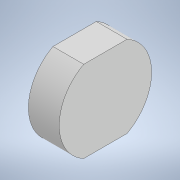
# Autodesk Inventor part: 711117
Saved by Autodesk Inventor 2022 (Build 260153000, 153)
## iProperties
Created: 2021-10-21
Part Number: 711117
Material: Типовые
Document SubType Name: Modeling
Designer: RaNSiD
Density: 1 g/cm^3
Appearance: По умолчанию
Author: RaNSiD
Autodesk Inventor part; units mm, degrees
ref_plane "YZ Plane" through (0, 0, 0) normal (1, 0, 0) x (0, 1, 0)
ref_plane "XZ Plane" through (0, 0, 0) normal (0, 1, 0) x (-1, 0, 0)
ref_plane "XY Plane" through (0, 0, 0) normal (0, 0, 1) x (1, 0, 0)
sketch "Эскиз1" plane through (0, 0, 0) normal (0, 0, 1) x (1, 0, 0)
  line L0 (0, 0) -> (20, 0)
  line L1 (20, 0) -> (20, 30)
  line L2 (20, 30) -> (0, 30)
  line L3 (0, 30) -> (0, 0)
  dimension "d0" = 20
  dimension "d1" = 30
  constraints: 8 end point, 2 parallel, 1 horizontal, 1 perpendicular
  measures "d0" distance of L2.end L1.end
  measures "d1" distance of L1.end L0.end
revolve "Вращение1" add sketch "Эскиз1" angle 360 about axis through (0, 0, 0) along (1, 0, 0)
sketch "Эскиз2" plane through (0, 0, 0) normal (0, 0, 1) x (1, 0, 0)
  line L0 (0, -30) -> (0, 30) construction
  line L1 (0, 20.647) -> (0, 23.353)
  line L2 (0, 23.353) -> (4, 24.5)
  line L3 (4, 24.5) -> (4, 19.5)
  line L4 (4, 19.5) -> (0, 20.647)
  line L5 (4, 22) -> (0, 22) construction
  line L6 (0, 0) -> (20.0289, 0)
  dimension "d3" = 74
  dimension "d4" = 74
  dimension "d5" = 5
  dimension "d6" = 4
  dimension "d7" = 22
  constraints: 12 end point, 2 midpoint, 2 point on line, 1 horizontal, 1 parallel
  measures "d3" angle of L3 L4
  measures "d4" angle of L2 L3
  measures "d5" distance of L2.end L3.end
  measures "d6" distance between parallel lines of L0 L3
  measures "d7" distance of L6.start L5.end
revolve "Вращение2" cut sketch "Эскиз2" angle 360 about axis through (0, 0, 0) along (1, 0, 0)
sketch "Эскиз3" plane through (0, 0, 0) normal (-1, 0, 0) x (0, 0, 1)
  line L0 (-30, -26.5) -> (-30, 26.5)
  line L1 (-30, 26.5) -> (30, 26.5)
  line L2 (30, 26.5) -> (30, -26.5)
  line L3 (30, -26.5) -> (-30, -26.5)
  point P0 (0, 0)
  point P1 (-30, 0)
  point P2 (30, 0)
  point P3 (0, 26.5)
  dimension "d9" = 53
  dimension "d10" = 60
  constraints: 8 end point, 3 midpoint, 2 horizontal alignment, 2 parallel, 1 perpendicular, 1 vertical, 1 vertical alignment
  measures "d9" distance of L1.end L2.end
  measures "d10" distance of L0.end L1.end
extrude "Выдавливание1" cut sketch "Эскиз3" against normal blind 20 keep common part
